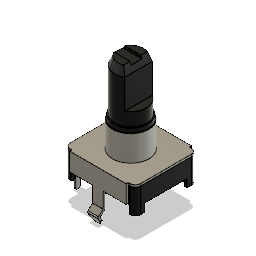
rotaryEncoder (Autodesk Fusion 360 design; units mm, degrees)
Autodesk Fusion 360 part; units mm, degrees
sketch "Sketch1" plane through (0, 0, 0) normal (0, 1, 0) x (1, 0, 0) in component "Plastic Body"
  line L0 (0, 0) -> (1.3, 0)
  line L1 (13.25, -1.8) -> (13.25, -9.7)
  line L2 (12, -11.5) -> (1.3, -11.5)
  line L3 (0, -1.8) -> (0, 0)
  line L4 (0.6, -1.8) -> (12.65, -1.8) construction
  line L5 (1.3, -1.8) -> (1.3, -10.9) construction
  line L6 (1.3, -0.6) -> (1.3, -1.8) construction
  line L7 (1.3, 0) -> (12, 0)
  line L8 (0, -9.7) -> (0, -1.8)
  line L9 (0.6, -1.8) -> (0.6, -0.6)
  line L10 (0.6, -0.6) -> (1.3, -0.6)
  line L11 (1.3, 0) -> (1.3, -0.6)
  line L12 (0, -1.8) -> (0.6, -1.8)
  line L13 (12, -0.6) -> (12, -10.9) construction
  line L14 (13.25, 0) -> (13.25, -1.8)
  line L15 (12, 0) -> (13.25, 0)
  line L16 (13.25, -9.7) -> (13.25, -11.5)
  line L17 (13.25, -11.5) -> (12, -11.5)
  line L18 (1.3, -11.5) -> (0, -11.5)
  line L19 (0, -11.5) -> (0, -9.7)
  line L20 (12, -0.6) -> (12.65, -0.6)
  line L21 (12.65, -0.6) -> (12.65, -1.8)
  line L22 (12.65, -9.7) -> (12.65, -10.9)
  line L23 (12.65, -10.9) -> (12, -10.9)
  line L24 (1.3, -10.9) -> (0.6, -10.9)
  line L25 (0.6, -10.9) -> (0.6, -9.7)
  line L26 (0.6, -9.7) -> (0, -9.7)
  line L27 (1.3, -9.7) -> (0.6, -9.7) construction
  line L28 (1.3, -10.9) -> (1.3, -11.5)
  line L29 (12, -10.9) -> (12, -11.5)
  line L30 (13.25, -9.7) -> (12.65, -9.7)
  line L31 (12, -9.7) -> (1.3, -9.7) construction
  line L32 (12.65, -9.7) -> (12, -9.7) construction
  line L33 (12.65, -1.8) -> (13.25, -1.8)
  line L34 (12, 0) -> (12, -0.6)
  dimension "d1" = 13.25
  dimension "d2" = 11.5
  dimension "d3" = 1.3
  dimension "d4" = 1.8
  dimension "d5" = 0.6
  dimension "d6" = 0.6
  dimension "d7" = 0.6
  dimension "d8" = 0.6
  measures "d1" distance of L0.start
  measures "d2" distance of L0.start
  measures "d4" distance of L0.start
  measures "d5" distance of L3
  measures "d6" distance of L15
  measures "d7" distance of L16
  measures "d8" distance of L18
extrude "Extrude1" add sketch "Sketch1" along normal blind 3.2 contours L1 L2 L7 L8 L9 L10 L11 L12 L20 L21 L22 L23 L24 L25 L26 L28 L29 L30 L33 L34 makes body 1 in component "Plastic Body"
extrude "Extrude2" add sketch "Sketch1" along normal up to surface (3.2 mm away) and the other way blind 1.5 contours L0 L3 L9 L10 L11 L12 | L14 L15 L20 L21 L33 L34 | L18 L19 L24 L25 L26 L28 | L16 L17 L22 L23 L29 L30 bodies 1 in component "Plastic Body"
fillet "Fillet1" radius 1 8 edges at (13.25, 0.85, 11.5) (0.6, -0.75, 0.6) (13.25, 0.85, 0) (0, 0.85, 11.5) (0, 0.85, 0) (0.6, -0.75, 10.9) (12.65, -0.75, 10.9) (12.65, -0.75, 0.6) on bodies 1 in component "Plastic Body"
hole "Hole1" at (6.625, 3.2, 5.75) direction (0, -1, 0) diameter 6.5 depth 3.2 tip angle 118 bodies 1 in component "Plastic Body"
sketch "Sketch1 (2)" plane through (0, 3.2, 0) normal (0, 1, 0) x (-1, 0, 0) in component "Metal Cover"
  circle A0 centre (-6.625, 5.75) radius 3.25
  arc A1 (-1, 0) -> (0, 1) centre (-1, 1) ccw
  line L0 (0, 1) -> (0, 10.5)
  arc A2 (0, 10.5) -> (-1, 11.5) centre (-1, 10.5) ccw
  line L1 (-1, 11.5) -> (-12.25, 11.5)
  arc A3 (-12.25, 11.5) -> (-13.25, 10.5) centre (-12.25, 10.5) ccw
  line L2 (-13.25, 10.5) -> (-13.25, 1)
  arc A4 (-13.25, 1) -> (-12.25, 0) centre (-12.25, 1) ccw
  line L3 (-12.25, 0) -> (-1, 0)
  circle A5 centre (-6.625, 5.75) radius 3.4
  line L4 (-6.625, 0) -> (-6.625, -0.4) construction
  line L5 (-1.325, -0.4) -> (-11.925, -0.4)
  line L6 (-1.325, -0.4) -> (-1.325, 0)
  line L7 (-11.925, -0.4) -> (-11.925, 0)
  line L8 (-6.625, 11.5) -> (-6.625, 11.9) construction
  line L9 (-4.625, 11.9) -> (-1.325, 11.9)
  line L10 (-1.325, 11.9) -> (-11.925, 11.9)
  line L11 (-11.925, 11.9) -> (-11.925, 11.5)
  line L12 (-1.325, 11.9) -> (-1.325, 11.5)
  dimension "d20" = 6.8
  dimension "d21" = 0.4
  dimension "d22" = 10.6
  dimension "d23" = 0.4
  dimension "d24" = 10.6
  measures "d20" diameter of A5
extrude "Extrude1'" add sketch "Sketch1 (2)" along normal blind 0.4 separate body contours A1 L0 A2 L1 A3 L2 A4 L3 | L3 L5 L6 L7 | L1 L9 L10 L11 L12 | A5 makes body 2 in component "Metal Cover"
extrude "Extrude2'" add sketch "Sketch1 (2)" along normal blind 5.2 contours A5 bodies 2 in component "Metal Cover"
extrude "Extrude3" add sketch "Sketch1 (2)" against normal blind 3 contours L3 L5 L6 L7 | L1 L9 L10 L11 L12 bodies 2 in component "Metal Cover"
sketch "Sketch2" plane through (0, 0.2, 0) normal (0, -1, 0) x (1, 0, 0) in component "Metal Cover"
  line L0 (11.925, 11.9) -> (1.325, 11.9)
  line L1 (1.325, 11.9) -> (1.325, 11.5)
  line L2 (1.325, 11.5) -> (11.925, 11.5)
  line L3 (11.925, 11.5) -> (11.925, 11.9)
  line L4 (5.625, 11.9) -> (7.625, 11.9)
  line L5 (5.625, 11.9) -> (5.625, 11.5)
  line L6 (7.625, 11.9) -> (7.625, 11.5)
  line L7 (5.625, -0.4) -> (7.625, -0.4)
  line L8 (1.3, 0) -> (12, 0)
  line L9 (7.625, -0.4) -> (7.625, 0)
  line L10 (5.625, -0.4) -> (5.625, 0)
  dimension "d31" = 2
  dimension "d32" = 2
extrude "Extrude4" add sketch "Sketch2" along normal blind 2.9 contours L0 L2 L4 L5 L6 | L7 L8 L9 L10 bodies 2 in component "Metal Cover"
sketch "Sketch3" plane through (5.625, 0, 0) normal (-1, 0, 0) x (0, 0, 1) in component "Metal Cover"
  line L0 (11.9, 0.2) -> (11.5, 0.2)
  line L1 (11.5, 0.2) -> (11.5, -2.7)
  line L2 (11.5, -2.7) -> (11.9, -2.7)
  line L3 (11.9, -2.7) -> (11.9, 0.2)
  line L4 (11.9, -2.7) -> (12.9725, -3.5999)
  line L5 (11.9, -2.7) -> (13.3, -2.7) construction
  line L6 (11.9, -2.7) -> (11.6429, -3.0064) construction
  line L7 (11.6429, -3.0064) -> (12.4582, -3.6906)
  line L8 (12.9725, -3.5999) -> (11.9725, -5.332)
  line L9 (12.9725, -3.5999) -> (14.9725, -3.5999) construction
  line L10 (11.9725, -5.332) -> (11.6261, -5.132)
  line L11 (11.6261, -5.132) -> (12.4582, -3.6906)
  line L12 (11.6429, -3.0064) -> (11.5, -2.8865)
  line L13 (11.5, -2.7) -> (11.5, -2.8865)
  dimension "d35" = 40
  dimension "d36" = 1.4
  dimension "d37" = 0.4
  dimension "d38" = 120
  dimension "d39" = 2
  dimension "d40" = 0.4
  measures "d35" angle of L4 L5
  measures "d38" angle of L8 L9
extrude "Extrude5" add sketch "Sketch3" against normal blind 2 contours L2 L4 L7 L8 L10 L11 L12 L13 bodies 2 in component "Metal Cover"
fillet "Fillet1'" radius 0.25 2 edges at (6.625, -2.8865, 11.5) (6.625, -3.5999, 12.9725) on bodies 2 in component "Metal Cover"
fillet "Fillet2" radius 1 2 edges at (5.625, -5.232, 11.7993) (7.625, -5.232, 11.7993) on bodies 2 in component "Metal Cover"
ref_plane "WorkPlane1" through (6.625, 0.215, 5.75) normal (0, 0, -1) x (1, 0, 0) in component "Metal Cover"
mirror "Mirror1" about plane through (6.625, 0.215, 5.75) normal (0, 0, -1) of "Extrude5", "Fillet1'", "Fillet2" in component "Metal Cover"
sketch "Sketch1 (3)" plane through (0, 0, 0) normal (0, 1, 0) x (1, 0, 0) in component "Shaft"
  circle A0 centre (6.625, -5.75) radius 3
  circle A1 centre (6.625, -5.75) radius 3.2497
  dimension "d46" = 6
  dimension "d47" = 0.2497
  measures "d46" diameter of A0
extrude "Extrude1''" add sketch "Sketch1 (3)" along normal blind 9.2 and the other way blind 0.5 separate body contours A0 | A1 makes body 3 in component "Shaft"
extrude "Extrude2''" add sketch "Sketch1 (3)" along normal blind 18.7 contours A0 bodies 3 in component "Shaft"
sketch "Sketch2 (2)" plane through (0, 18.7, 0) normal (0, 1, 0) x (-1, 0, 0) in component "Shaft"
  circle A0 centre (-6.625, 5.75) radius 3
  line L0 (-3.625, 5.75) -> (-8.125, 5.75) construction
  line L1 (-8.125, 4.75) -> (-8.125, 6.75)
  circle A1 centre (-6.625, 5.75) radius 3
  line L2 (-8.125, 6.75) -> (-8.125, 8.3481)
  line L3 (-8.125, 3.1519) -> (-8.125, 4.75)
  line L4 (-8.125, 4.75) -> (-3.7966, 4.75)
  line L5 (-8.125, 6.75) -> (-3.7966, 6.75)
  dimension "d54" = 4.5
  dimension "d55" = 2
extrude "Extrude3'" cut sketch "Sketch2 (2)" against normal blind 7 contours A0 L1 A1 L2 L3 bodies 3 in component "Shaft"
extrude "Extrude4'" cut sketch "Sketch2 (2)" against normal blind 0.5 contours A0 L1 A1 L4 L5 bodies 3 in component "Shaft"
chamfer "Chamfer1" distance 0.5 angle 45 1 edges at (3.5953, -0.5, 4.5749) on bodies 3 in component "Shaft"
hole "Hole1'" at (6.625, -0.5, 5.75) direction (0, 1, 0) diameter 4 depth 7.5 tip angle 180 bodies 3 in component "Shaft"
chamfer "Chamfer2" distance 0.6 distance2 1.5 4 edges at (5.5859, 18.7, 8.5643) (5.5859, 18.7, 2.9357) (8.125, 18.7, 7.549) (8.125, 18.7, 3.951) measured on face at (5.298, 18.7, 6.8838) measured on face at (5.298, 18.7, 4.6162) measured on face at (5.298, 18.7, 6.8838) measured on face at (5.298, 18.7, 4.6162) on bodies 3 in component "Shaft"
sketch "Sketch1 (4)" plane through (0, 0, 0) normal (-1, 0, 0) x (0, 0, 1) in component "Pin"
  line L0 (1, 3.2) -> (1, -1.5)
  line L1 (1, -1.5) -> (1.8, -1.5)
  line L2 (1.8, -1.5) -> (1.8, 0)
  line L3 (1.8, 0) -> (9.7, 0)
  line L4 (9.7, 0) -> (9.7, -1.5)
  line L5 (9.7, -1.5) -> (10.5, -1.5)
  line L6 (10.5, -1.5) -> (10.5, 3.2)
  line L7 (10.5, 3.2) -> (1, 3.2)
  line L8 (5.75, 0) -> (5.75, 0.8) construction
  line L9 (5.75, 0.95) -> (5.75, 0.65) construction
  line L10 (5, 0.95) -> (6.5, 0.95)
  line L11 (6.5, 0.95) -> (6.5, 0.65)
  line L12 (6.5, 0.65) -> (5, 0.65)
  line L13 (5, 0.65) -> (5, 0.95)
  line L14 (5.75, 0.95) -> (8.29, 0.95) construction
  line L15 (5.75, 0.95) -> (3.21, 0.95) construction
  dimension "d66" = 0.8
  dimension "d67" = 0.3
  dimension "d68" = 1.5
  dimension "d84" = 2.54
  dimension "d85" = 2.54
extrude "Extrude1'''" add sketch "Sketch1 (4)" along normal blind 0.7 separate body contours L10 L11 L12 L13 makes body 4 in component "Pin"
sketch "Sketch2 (3)" plane through (0, 0, 6.5) normal (0, 0, 1) x (1, 0, 0) in component "Pin"
  line L0 (0, 0.65) -> (0, 0.95)
  line L1 (0, 0.95) -> (-0.7, 0.95)
  line L2 (-0.7, 0.95) -> (-0.7, 0.65)
  line L3 (-0.7, 0.65) -> (0, 0.65)
  line L4 (-0.7, 0.65) -> (-0.7, -5.35)
  line L5 (-0.7, 0.95) -> (-1, 0.95)
  line L6 (-1, 0.95) -> (-1, -5.35)
  line L7 (-1, -5.35) -> (-0.7, -5.35)
  dimension "d71" = 6
  dimension "d72" = 0.3
  measures "d71" distance of origin
extrude "Extrude2'''" add sketch "Sketch2 (3)" against normal blind 1.5 contours L2 L4 L5 L6 L7 bodies 4 in component "Pin"
sketch "Sketch3 (2)" plane through (-1, 0, 0) normal (-1, 0, 0) x (0, 0, 1) in component "Pin"
  line L0 (6.5, -5.35) -> (6.5, 0.95)
  line L1 (6.5, 0.95) -> (5, 0.95)
  line L2 (5, 0.95) -> (5, -5.35)
  line L3 (5, -5.35) -> (6.5, -5.35)
  line L4 (5.75, 0.95) -> (5.75, -1.05) construction
  line L5 (5.3, -1.05) -> (6.2, -1.05)
  line L6 (5.3, -1.05) -> (5, -1.05)
  line L7 (5.3, -1.05) -> (5.3, -5.35)
  line L8 (6.2, -1.05) -> (6.5, -1.05)
  line L9 (6.2, -1.05) -> (6.2, -5.35)
  dimension "d75" = 2
  dimension "d76" = 0.9
extrude "Extrude3''" cut sketch "Sketch3 (2)" against normal through all contours L0 L3 L8 L9 | L2 L3 L6 L7 bodies 4 in component "Pin"
fillet "Fillet2'" radius 0.25 1 edges at (-1, 0.95, 5.75) on bodies 4 in component "Pin"
fillet "Fillet1''" radius 0.3 2 edges at (-0.85, -5.35, 5.3) (-0.85, -5.35, 6.2) on bodies 4 in component "Pin"
other "PathPattern1" in component "Pins"
sketch "Sketch2 (4)" plane through (0, 0, 0) normal (-1, 0, 0) x (0, 0, 1) in component "Plastic Body"
  line L0 (1, 3.2) -> (1, -1.5)
  line L1 (1, -1.5) -> (1.8, -1.5)
  line L2 (1.8, -1.5) -> (1.8, 0)
  line L3 (1.8, 0) -> (9.7, 0)
  line L4 (9.7, 0) -> (9.7, -1.5)
  line L5 (9.7, -1.5) -> (10.5, -1.5)
  line L6 (10.5, -1.5) -> (10.5, 3.2)
  line L7 (10.5, 3.2) -> (1, 3.2)
  line L8 (6.5, 0.95) -> (5, 0.95)
  line L9 (5.75, 0.95) -> (8.29, 0.95) construction
  line L10 (5.75, 0.95) -> (3.21, 0.95) construction
  dimension "d90" = 2.54
  dimension "d91" = 2.54
component "Rotary Encoder" placed x (1, 0, 0) y (0, 1, 0) z (0, 0, 1) at (0, 0, 0)
component "Plastic Body" placed x (1, 0, 0) y (0, 1, 0) z (0, 0, 1) at (0, 0, 0) in component "Rotary Encoder"
component "Metal Cover" placed x (1, 0, 0) y (0, 1, 0) z (0, 0, 1) at (0, 0, 0) in component "Rotary Encoder"
component "Shaft" placed x (1, 0, 0) y (0, 1, 0) z (0, 0, 1) at (0, 0, 0) in component "Rotary Encoder"
component "Pins" placed x (1, 0, 0) y (0, 1, 0) z (0, 0, 1) at (0, 0, 0) in component "Rotary Encoder"
component "Pin" placed x (1, 0, 0) y (0, 1, 0) z (0, 0, 1) at (0, 0, 0) in component "Pins"
component "Pin" placed x (1, 0, 0) y (0, 1, 0) z (0, 0, 1) at (0, 0, 2.54) in component "Pins"
component "Pin" placed x (1, 0, 0) y (0, 1, 0) z (0, 0, 1) at (0, 0, -2.54) in component "Pins"
equation "d9 = 3.6 mm - 0.4 mm"
equation "d27 = 0.4 mm + 4.8 mm"
equation "d48 = 8.40 mm + 0.8 mm"
equation "d52 = 8.40 mm + 10.3 mm"
equation "d69 = 1 mm - 0.3 mm"
